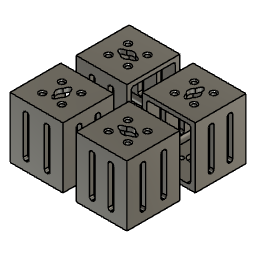
non_rotating_motor_stand_set v1 (Autodesk Fusion 360 design; units mm, degrees)
Autodesk Fusion 360 part; units mm, degrees
sketch "Sketch1" plane through (0, 0, 0) normal (0, 0, 1) x (1, 0, 0)
  line L0 (-24, -23) -> (24, -23)
  line L1 (24, -23) -> (24, 23)
  line L2 (24, 23) -> (-24, 23)
  line L3 (-24, 23) -> (-24, -23)
  dimension "d1" = 48
  dimension "d2" = 46
  dimension "d3" = 24
  dimension "d4" = 23
  constraint horizontal L0
  constraint vertical L1
  constraint horizontal L2
  constraint vertical L3
  measures "d1" distance of L1.end L2.end
  measures "d2" distance of L0.start L2.end
  measures "d3" distance of origin L1
  measures "d4" distance of origin L0
extrude "Extrude1" add sketch "Sketch1" along normal blind 55 makes body 1
sketch "Sketch2" plane through (0, -23, 0) normal (0, -1, 0) x (1, 0, 0)
  line L0 (-24, 0) -> (24, 0)
  line L1 (24, 0) -> (24, 55)
  line L2 (24, 55) -> (-24, 55)
  line L3 (-24, 55) -> (-24, 0)
  line L4 (-20, 51) -> (20, 51)
  line L5 (20, 51) -> (20, 4)
  line L6 (20, 4) -> (-20, 4)
  line L7 (-20, 4) -> (-20, 51)
  dimension "d7" = 40
  dimension "d8" = 20
  dimension "d10" = 4
  dimension "d58" = 4
  constraint horizontal L4
  constraint vertical L5
  constraint horizontal L6
  constraint vertical L7
  measures "d7" distance of L4.start L4.end
  measures "d8" distance of origin L7
  measures "d10" distance of L2 L4
  measures "d58" distance of L0 L6
extrude "Extrude2" cut sketch "Sketch2" against normal blind 42 contours L4 L5 L6 L7 bodies 1
sketch "Sketch4" plane through (0, 0, 55) normal (0, 0, 1) x (-1, 0, 0)
  line L0 (24, -23) -> (24, 23)
  line L1 (24, 23) -> (-24, 23)
  line L2 (-24, 23) -> (-24, -23)
  line L3 (-24, -23) -> (24, -23)
  circle A0 centre (0, 0) radius 5
  dimension "d23" = 10
  constraint coincident A0.centre origin
  measures "d23" diameter of A0
hole "Hole1" at (0, 0, 55) direction (0, 0, -1) diameter 10 depth 4 tip angle 118 bodies 1
sketch "Sketch5" plane through (0, 0, 55) normal (0, 0, 1) x (-1, 0, 0)
  circle A0 centre (0, 0) radius 5
  line L0 (24, -23) -> (24, 23)
  line L1 (24, 23) -> (-24, 23)
  line L2 (-24, 23) -> (-24, -23)
  line L3 (-24, -23) -> (24, -23)
  circle A1 centre (-8.8388, -8.8388) radius 1.5
  point P0 (8.8388, -8.8388)
  point P1 (8.8388, 8.8388)
  point P2 (-8.8388, 8.8388)
  dimension "d27" = 12.5
  dimension "d28" = 3
  dimension "d30" = 360
  measures "d27" distance of A0.centre A1.centre
  measures "d28" diameter of A1
hole "Hole2" at (8.8388, 8.8388, 55) at (-8.8388, 8.8388, 55) at (-8.8388, -8.8388, 55) at (8.8388, -8.8388, 55) direction (0, 0, -1) diameter 4 depth 4 tip angle 118 countersink diameter 6 countersink angle 90 bodies 1
sketch "Sketch7" plane through (0, 0, 0) normal (0, 0, -1) x (1, 0, 0)
  line L0 (-24, 23) -> (-24, -23)
  line L1 (-24, -23) -> (24, -23)
  line L2 (24, -23) -> (24, 23)
  line L3 (24, 23) -> (-24, 23)
  circle A0 centre (0, 0) radius 5
  circle A1 centre (5.6569, -5.6569) radius 2
  circle A2 centre (6.7175, 6.7175) radius 2
  circle A3 centre (-6.7175, -6.7175) radius 2
  circle A4 centre (-5.6569, 5.6569) radius 2
  dimension "d45" = 10
  dimension "d67" = 4
  dimension "d68" = 4
  dimension "d69" = 9.5
  dimension "d70" = 8
  dimension "d71" = 17.3431
  dimension "d72" = 16.2825
  dimension "d74" = 360
  constraint coincident A0.centre origin
  measures "d45" diameter of A0
  measures "d67" diameter of A2
  measures "d68" diameter of A1
  measures "d69" distance of A0.centre A2.centre
  measures "d70" distance of A0.centre A1.centre
  measures "d71" distance of L1 A1.centre
  measures "d72" distance of L3 A2.centre
extrude "Extrude4" cut sketch "Sketch7" against normal blind 4 contours A0 | A1 | A2 | A3 | A4 bodies 1
sketch "Sketch8" plane through (0, 0, 55) normal (0, 0, 1) x (-1, 0, 0)
  circle A0 centre (0, 0) radius 5
  line L0 (24, -23) -> (24, 23)
  line L1 (24, 23) -> (-24, 23)
  line L2 (-24, 23) -> (-24, -23)
  line L3 (-24, -23) -> (24, -23)
  ellipse E0 centre (0, 0) end of major axis (0, 8.5421) minor radius 3.3168
  line L4 (0, -8.5421) -> (0, 8.5421)
  line L5 (3.3168, 0) -> (-3.3168, 0)
  circle A1 centre (8.8388, 8.8388) radius 3
  circle A2 centre (-8.8388, -8.8388) radius 3
  circle A3 centre (8.8388, -8.8388) radius 3
  circle A4 centre (-8.8388, 8.8388) radius 3
  constraint coincident E0 L4.start
  constraint coincident E0 L4.end
  constraint coincident E0 L5.start
  constraint coincident E0 L5.end
  constraint concentric A0 E0
  constraint vertical L4
extrude "Extrude5" cut sketch "Sketch8" against normal blind 4 contours A0 E0 L4 | A0 E0 L4 | A0 E0 L4 | A0 E0 L4 bodies 1
sketch "Sketch3" plane through (24, 0, 0) normal (1, 0, 0) x (0, 1, 0)
  line L0 (-21, 0) -> (23, 0)
  line L1 (23, 0) -> (23, 50)
  line L2 (23, 50) -> (-21, 50)
  line L3 (-11, 47) -> (-6, 47)
  line L4 (-6, 47) -> (-6, 8)
  line L5 (-6, 8) -> (-11, 8)
  line L6 (-11, 8) -> (-11, 47)
  line L7 (6, 47) -> (11, 47)
  line L8 (11, 47) -> (11, 8)
  line L9 (11, 8) -> (6, 8)
  line L10 (6, 8) -> (6, 47)
  line L11 (-23, 0) -> (23, 0)
  line L12 (23, 0) -> (23, 55)
  line L13 (23, 55) -> (-23, 55)
  line L14 (-23, 55) -> (-23, 0)
  line L15 (-23, 51) -> (-23, 4)
  point P0 (-23, 55)
  point P1 (23, 55)
  dimension "d16" = 8
  dimension "d20" = 12
  dimension "d60" = 8
  dimension "d75" = 5
  dimension "d76" = 5
  dimension "d97" = 12
  dimension "d100" = 8
  dimension "d101" = 8
  constraint horizontal L3
  constraint vertical L4
  constraint horizontal L5
  constraint vertical L6
  constraint horizontal L7
  constraint vertical L8
  constraint horizontal L9
  constraint vertical L10
  measures "d16" distance of L0 L5
  measures "d20" distance of L1 L8
  measures "d60" distance of L0 L9
  measures "d75" distance of L3.start L3.end
  measures "d76" distance of L7.start L7.end
  measures "d97" distance of L5.end L15
  measures "d100" vertical distance of L3.start P0
  measures "d101" vertical distance of L7.end P1
extrude "Extrude6" cut sketch "Sketch3" against normal blind 48 contours L3 L4 L5 L6 | L7 L8 L9 L10 bodies 1
sketch "Sketch9" plane through (0, 23, 0) normal (0, 1, 0) x (-1, 0, 0)
  line L0 (-24, 0) -> (24, 0)
  line L1 (24, 0) -> (24, 55)
  line L2 (24, 55) -> (-24, 55)
  line L3 (-24, 55) -> (-24, 0)
  line L4 (-12, 47) -> (-7, 47)
  line L5 (-7, 47) -> (-7, 8)
  line L6 (-7, 8) -> (-12, 8)
  line L7 (-12, 8) -> (-12, 47)
  line L8 (7, 47) -> (12, 47)
  line L9 (12, 47) -> (12, 8)
  line L10 (12, 8) -> (7, 8)
  line L11 (7, 8) -> (7, 47)
  line L12 (-24, 0) -> (24, 0)
  dimension "d79" = 8
  dimension "d80" = 8
  dimension "d81" = 8
  dimension "d82" = 8
  dimension "d83" = 12
  dimension "d84" = 12
  dimension "d85" = 5
  dimension "d86" = 5
  constraint horizontal L4
  constraint vertical L5
  constraint horizontal L6
  constraint vertical L7
  constraint horizontal L8
  constraint vertical L9
  constraint horizontal L10
  constraint vertical L11
  measures "d79" distance of L2 L4
  measures "d80" distance of L2 L8
  measures "d81" distance of L10 L12
  measures "d82" distance of L6 L12
  measures "d83" distance of L3 L7
  measures "d84" distance of L1 L9
  measures "d85" distance of L4.start L4.end
  measures "d86" distance of L8.start L8.end
extrude "Extrude7" cut sketch "Sketch9" against normal blind 44 contours L4 L5 L6 L7 | L8 L9 L10 L11 bodies 1
fillet "Fillet2" radius 3.5 3 edges at (0, 19, 4) (-20, -2, 4) (20, -2, 4) on bodies 1
fillet "Fillet3" radius 2 24 edges at (22, 11, 8) (22, -6, 8) (-22, 11, 8) (-22, -6, 8) (22, 6, 8) (22, -11, 8) (22, -11, 47) (22, 6, 47) (22, 11, 47) (22, -6, 47) (-22, -6, 47) (-22, -11, 47) (-22, 6, 47) (-22, 11, 47) (-22, -11, 8) (-22, 6, 8) (-7, 21, 8) (12, 21, 8) (7, 21, 8) (-12, 21, 8) (12, 21, 47) (-7, 21, 47) (7, 21, 47) (-12, 21, 47) on bodies 1
fillet "Fillet4" radius 2 3 edges at (-20, -2, 51) (0, 19, 51) (20, -2, 51) on bodies 1
move_body "Move1" bodies 1 to x (1, 0, 0) y (0, 1, 0) z (0, 0, 1) at (30, 30, 0)
pattern_circular "C-Pattern1" count 4 over 360 about axis through (0, 0, 1.75) along (0, 0, 1) of bodies 1 makes body 2 at (-53, 32.3333, 33.3333) makes body 3 at (-32.3333, -53, 33.3333) makes body 4 at (53, -32.3333, 21.6667)
